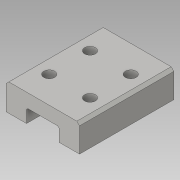
# Autodesk Inventor part: MGN Block
Saved by Autodesk Inventor 2016 (Build 200138000, 138)
## iProperties
Created: 2017-05-18
Part Number: MGN Block
Material: Generic
Document SubType Name: Modeling
Designer: 31745
Density: 1 g/cm^3
Appearance: Default
Author: 31745
Autodesk Inventor part; units mm, degrees
ref_plane "YZ Plane" through (0, 0, 0) normal (1, 0, 0) x (0, 1, 0)
ref_plane "XZ Plane" through (0, 0, 0) normal (0, 1, 0) x (-1, 0, 0)
ref_plane "XY Plane" through (0, 0, 0) normal (0, 0, 1) x (1, 0, 0)
sketch "Sketch1" plane through (0, 0, 0) normal (0, 0, 1) x (1, 0, 0)
  line L0 (0, 0) -> (27, 0)
  line L1 (27, 0) -> (27, 10)
  line L2 (27, 10) -> (0, 10)
  line L3 (0, 10) -> (0, 0)
  line L4 (7.5, 0) -> (19.5, 0)
  line L5 (19.5, 0) -> (19.5, 5)
  line L6 (19.5, 5) -> (7.5, 5)
  line L7 (7.5, 5) -> (7.5, 0)
  point P0 (13.5, 5)
  point P1 (13.5, 10)
  dimension "d0" = 27
  dimension "d1" = 10
  dimension "d2" = 5
  dimension "d3" = 12
  constraints: 16 end point, 4 parallel, 2 horizontal, 2 midpoint, 2 perpendicular, 1 point on line, 1 vertical alignment
  measures "d0" distance of L2.end L1.end
  measures "d1" distance of L1.end L0.end
  measures "d2" distance of L4.end L5.end
  measures "d3" distance of L5.end L6.end
extrude "Extrusion1" add sketch "Sketch1" along normal blind 34.7 contours L3 L2 L1 L0 L5 L6 L7
chamfer "Chamfer1" distance 1 angle 45 2 edges at (27, 10, 17.35) (0, 10, 17.35)
chamfer "Chamfer2" distance 0.5 angle 45 2 edges at (7.5, 5, 17.35) (19.5, 5, 17.35)
sketch "Sketch2" plane through (1, 10, 0) normal (0, 1, 0) x (1, 0, 0)
  line L0 (18, -34.7) -> (18, 0) projected
  line L1 (-1, 0) -> (-1, -34.7) projected
  line L2 (25, 0) -> (0, 0) projected
  line L3 (5, -9.85) -> (20, -9.85)
  line L4 (20, -9.85) -> (20, -24.85)
  line L5 (20, -24.85) -> (5, -24.85)
  line L6 (5, -24.85) -> (5, -9.85)
  line L7 (25, 0) -> (25, -34.7) projected
  point P0 (-1, -17.35)
  point P1 (12.5, 0)
  point P2 (12.5, -9.85)
  point P3 (12.5, 0)
  point P4 (20, -17.35)
  point P5 (25, -17.35)
  dimension "d12" = 15
  dimension "d13" = 15
  constraints: 8 end point, 6 midpoint, 4 coincident, 2 parallel, 1 horizontal, 1 horizontal alignment, 1 perpendicular, 1 vertical alignment
  measures "d12" distance of L3.end L4.end
  measures "d13" distance of L3.start L3.end
hole "Hole1" at (21, 10, 9.85) at (21, 10, 24.85) at (6, 10, 24.85) at (6, 10, 9.85) direction (0, -1, 0) diameter 4 end through all
body "Solid1"
